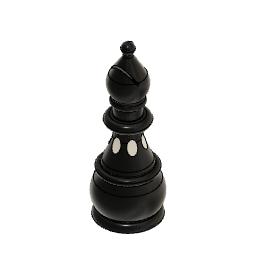
Bishop (Autodesk Fusion 360 design; units mm, degrees)
Autodesk Fusion 360 part; units mm, degrees
(part 1 of 2)
sketch "Bishop" plane through (0, 0, 0) normal (1, 0, 0) x (0, 1, 0)
  spline S0 degree 3 poles (89.633726, 49.908438) (91.318246, 50.120516) (92.983019, 49.910348) (94.642058, 49.967669) knots 0 0 0 0 1 1 1 1
  spline S1 degree 3 poles (94.642058, 49.967669) (95.185947, 49.986137) (95.040743, 49.595738) (95.026729, 49.350542) knots 0 0 0 0 1 1 1 1
  spline S2 degree 3 poles (95.026729, 49.350542) (94.969414, 48.413708) (94.850321, 47.480061) (94.788545, 46.543228) knots 0 0 0 0 1 1 1 1
  spline S3 degree 3 poles (94.788545, 46.543228) (94.752239, 45.984058) (94.746515, 45.546527) (95.629848, 45.661163) knots 0 0 0 0 1 1 1 1
  spline S4 degree 3 poles (95.629848, 45.661163) (96.260983, 45.742682) (96.968548, 45.715933) (97.618789, 45.643968) knots 0 0 0 0 1 1 1 1
  spline S5 degree 3 poles (97.618789, 45.643968) (98.646062, 45.529968) (98.735855, 46.002527) (98.608483, 46.807529) knots 0 0 0 0 1 1 1 1
  spline S6 degree 3 poles (98.608483, 46.807529) (98.484289, 47.590879) (98.454358, 48.390147) (98.321894, 49.171583) knots 0 0 0 0 1 1 1 1
  spline S7 degree 3 poles (98.321894, 49.171583) (98.219993, 49.771514) (98.467098, 49.985501) (99.011618, 49.984864) knots 0 0 0 0 1 1 1 1
  spline S8 degree 3 poles (99.011618, 49.984864) (100.513355, 49.982955) (102.016365, 49.980404) (103.516828, 49.971488) knots 0 0 0 0 1 1 1 1
  spline S9 degree 3 poles (103.516828, 49.971488) (104.025684, 49.968942) (104.316733, 49.857488) (104.202733, 49.195144) knots 0 0 0 0 1 1 1 1
  spline S10 degree 3 poles (104.202733, 49.195144) (103.791319, 46.807524) (103.216226, 44.43328) (101.692197, 42.543053) knots 0 0 0 0 1 1 1 1
  spline S11 degree 3 poles (101.692197, 42.543053) (100.940055, 41.611316) (100.165621, 40.511441) (98.410414, 40.603148) knots 0 0 0 0 1 1 1 1
  spline S12 degree 3 poles (98.410414, 40.603148) (94.261848, 40.819681) (90.094818, 40.657287) (85.935436, 40.638172) knots 0 0 0 0 1 1 1 1
  spline S13 degree 3 poles (85.935436, 40.638172) (85.306206, 40.635626) (84.747673, 40.755991) (84.289127, 41.227277) knots 0 0 0 0 1 1 1 1
  spline S14 degree 3 poles (84.289127, 41.227277) (82.099571, 43.484974) (81.055749, 46.249622) (80.711202, 49.320601) knots 0 0 0 0 1 1 1 1
  spline S15 degree 3 poles (80.711202, 49.320601) (80.677452, 49.61547) (80.535426, 50.020519) (81.126436, 50.01033) knots 0 0 0 0 1 1 1 1
  spline S16 degree 3 poles (81.126436, 50.01033) (82.665752, 49.983581) (84.206331, 49.988037) (85.746278, 49.984218) knots 0 0 0 0 1 1 1 1
  spline S17 degree 3 poles (85.746278, 49.984218) (86.327736, 49.982308) (86.595861, 49.77405) (86.497779, 49.124447) knots 0 0 0 0 1 1 1 1
  spline S18 degree 3 poles (86.497779, 49.124447) (86.358308, 48.198438) (86.310535, 47.258422) (86.213736, 46.326048) knots 0 0 0 0 1 1 1 1
  spline S19 degree 3 poles (86.213736, 46.326048) (86.173611, 45.952208) (86.203542, 45.58346) (86.677374, 45.62995) knots 0 0 0 0 1 1 1 1
  spline S20 degree 3 poles (86.677374, 45.62995) (87.675348, 45.7293) (88.681601, 45.46946) (89.679575, 45.733761) knots 0 0 0 0 1 1 1 1
  spline S21 degree 3 poles (89.679575, 45.733761) (89.932413, 45.80127) (90.126654, 45.768152) (90.090358, 46.115881) knots 0 0 0 0 1 1 1 1
  spline S22 degree 3 poles (90.090358, 46.115881) (89.957884, 47.366698) (90.020933, 48.639794) (89.633726, 49.908438) knots 0 0 0 0 1 1 1 1
  spline S23 degree 3 poles (34.222983, 55.82431) (32.279896, 55.735786) (30.397312, 57.485901) (30.278857, 59.490764) knots 0 0 0 0 1 1 1 1
  spline S24 degree 3 poles (30.278857, 59.490764) (30.143205, 61.784126) (31.853196, 63.806822) (33.99753, 63.887704) knots 0 0 0 0 1 1 1 1
  spline S25 degree 3 poles (33.99753, 63.887704) (36.27115, 63.973046) (38.379183, 62.435008) (38.342882, 59.572919) knots 0 0 0 0 1 1 1 1
  spline S26 degree 3 poles (38.342882, 59.572919) (38.32123, 57.901134) (36.937954, 55.866976) (34.222983, 55.82431) knots 0 0 0 0 1 1 1 1
  spline S27 degree 3 poles (-1.934587, 66.923013) (-1.384334, 66.299521) (-0.785039, 65.859444) (-0.062195, 65.572214) knots 0 0 0 0 1 1 1 1
  spline S28 degree 3 poles (-0.062195, 65.572214) (0.214844, 65.462038) (0.465768, 65.420003) (0.699499, 65.557564) knots 0 0 0 0 1 1 1 1
  spline S29 degree 3 poles (0.699499, 65.557564) (1.023028, 65.7499) (0.936415, 66.105271) (0.871454, 66.378488) knots 0 0 0 0 1 1 1 1
  spline S30 degree 3 poles (0.871454, 66.378488) (0.730069, 66.972686) (0.440932, 67.494281) (-0.037995, 67.904423) knots 0 0 0 0 1 1 1 1
  spline S31 degree 3 poles (-0.037995, 67.904423) (-0.447502, 68.255339) (-0.327771, 68.518998) (0.135233, 68.714521) knots 0 0 0 0 1 1 1 1
  spline S32 degree 3 poles (0.135233, 68.714521) (0.833241, 69.008753) (1.581561, 69.087725) (2.297402, 68.987739) knots 0 0 0 0 1 1 1 1
  spline S33 degree 3 poles (2.297402, 68.987739) (3.616356, 68.80241) (3.670489, 68.565493) (2.908795, 67.495554) knots 0 0 0 0 1 1 1 1
  spline S34 degree 3 poles (2.908795, 67.495554) (2.533045, 66.967589) (1.901268, 66.323077) (2.508206, 65.723151) knots 0 0 0 0 1 1 1 1
  spline S35 degree 3 poles (2.508206, 65.723151) (3.166089, 65.07227) (3.829069, 65.777284) (4.355762, 66.168321) knots 0 0 0 0 1 1 1 1
  spline S36 degree 3 poles (4.355762, 66.168321) (5.255658, 66.836398) (5.526324, 66.817288) (5.709107, 65.735886) knots 0 0 0 0 1 1 1 1
  spline S37 degree 3 poles (5.709107, 65.735886) (5.851765, 64.889487) (5.939017, 64.015066) (5.533331, 63.171217) knots 0 0 0 0 1 1 1 1
  spline S38 degree 3 poles (5.533331, 63.171217) (5.298966, 62.684013) (5.146114, 62.477033) (4.725783, 63.010727) knots 0 0 0 0 1 1 1 1
  spline S39 degree 3 poles (4.725783, 63.010727) (4.343663, 63.494112) (3.809964, 63.806812) (3.2215, 63.971126) knots 0 0 0 0 1 1 1 1
  spline S40 degree 3 poles (3.2215, 63.971126) (2.526038, 64.164735) (2.188499, 63.820189) (2.334344, 63.116447) knots 0 0 0 0 1 1 1 1
  spline S41 degree 3 poles (2.334344, 63.116447) (2.477002, 62.429265) (2.942554, 61.930598) (3.359703, 61.409003) knots 0 0 0 0 1 1 1 1
  spline S42 degree 3 poles (3.359703, 61.409003) (3.68578, 61.001408) (3.646291, 60.814169) (3.095402, 60.672148) knots 0 0 0 0 1 1 1 1
  spline S43 degree 3 poles (3.095402, 60.672148) (2.166847, 60.432049) (1.255489, 60.306587) (0.328207, 60.627567) knots 0 0 0 0 1 1 1 1
  spline S44 degree 3 poles (0.328207, 60.627567) (-0.281913, 60.839008) (-0.651295, 61.066371) (0.018053, 61.712792) knots 0 0 0 0 1 1 1 1
  spline S45 degree 3 poles (0.018053, 61.712792) (0.388711, 62.07071) (0.599512, 62.6025) (0.84853, 63.073781) knots 0 0 0 0 1 1 1 1
  spline S46 degree 3 poles (0.84853, 63.073781) (0.982272, 63.327256) (0.928138, 63.615118) (0.736442, 63.827195) knots 0 0 0 0 1 1 1 1
  spline S47 degree 3 poles (0.736442, 63.827195) (0.536466, 64.048825) (0.28936, 64.049462) (0.004681, 63.928455) knots 0 0 0 0 1 1 1 1
  spline S48 degree 3 poles (0.004681, 63.928455) (-0.576142, 63.68135) (-1.183716, 63.494112) (-1.608507, 62.980159) knots 0 0 0 0 1 1 1 1
  spline S49 degree 3 poles (-1.608507, 62.980159) (-1.946047, 62.571927) (-2.163858, 62.72732) (-2.298236, 63.152112) knots 0 0 0 0 1 1 1 1
  spline S50 degree 3 poles (-2.298236, 63.152112) (-2.696281, 64.412482) (-2.760606, 65.645457) (-1.934587, 66.923013) knots 0 0 0 0 1 1 1 1
  spline S51 degree 3 poles (135.600981, 40.433747) (133.48084, 41.948856) (131.880389, 43.867104) (130.776695, 46.222879) knots 0 0 0 0 1 1 1 1
  spline S52 degree 3 poles (130.776695, 46.222879) (130.465899, 46.885859) (130.146201, 47.600427) (129.560915, 48.05133) knots 0 0 0 0 1 1 1 1
  spline S53 degree 3 poles (129.560915, 48.05133) (128.941889, 48.527708) (128.596692, 48.92957) (128.911938, 49.784249) knots 0 0 0 0 1 1 1 1
  spline S54 degree 3 poles (128.911938, 49.784249) (129.168606, 50.479075) (128.70559, 51.170713) (128.159797, 51.512708) knots 0 0 0 0 1 1 1 1
  spline S55 degree 3 poles (128.159797, 51.512708) (127.687238, 51.80885) (127.289195, 51.243315) (126.961218, 50.86947) knots 0 0 0 0 1 1 1 1
  spline S56 degree 3 poles (126.961218, 50.86947) (126.623037, 50.48544) (126.252379, 50.418567) (125.714224, 50.510274) knots 0 0 0 0 1 1 1 1
  spline S57 degree 3 poles (125.714224, 50.510274) (122.957224, 50.980919) (120.330773, 50.530016) (117.857816, 49.214886) knots 0 0 0 0 1 1 1 1
  spline S58 degree 3 poles (117.857816, 49.214886) (115.538974, 47.98191) (114.006033, 46.068754) (112.929724, 43.706609) knots 0 0 0 0 1 1 1 1
  spline S59 degree 3 poles (112.929724, 43.706609) (111.550267, 40.681484) (110.908306, 37.485043) (110.693678, 34.205806) knots 0 0 0 0 1 1 1 1
  spline S60 degree 3 poles (110.693678, 34.205806) (110.458671, 30.60623) (110.608336, 27.006003) (111.310799, 23.459283) knots 0 0 0 0 1 1 1 1
  spline S61 degree 3 poles (111.310799, 23.459283) (111.687823, 21.556316) (112.158467, 19.674378) (113.022704, 17.900056) knots 0 0 0 0 1 1 1 1
  spline S62 degree 3 poles (113.022704, 17.900056) (113.319487, 17.288026) (113.674859, 16.981059) (114.204092, 16.876611) knots 0 0 0 0 1 1 1 1
  line L0 (114.204092, 16.876611) -> (129.580001, 16.876611)
  spline S63 degree 3 poles (129.580001, 16.876611) (129.992698, 16.962585) (130.1621, 17.234529) (130.216228, 17.738934) knots 0 0 0 0 1 1 1 1
  spline S64 degree 3 poles (130.216228, 17.738934) (130.427028, 19.65846) (130.655028, 21.575431) (130.904037, 23.489223) knots 0 0 0 0 1 1 1 1
  spline S65 degree 3 poles (130.904037, 23.489223) (130.976649, 24.044569) (130.811699, 24.4165) (130.39836, 24.803717) knots 0 0 0 0 1 1 1 1
  spline S66 degree 3 poles (130.39836, 24.803717) (128.511952, 26.564016) (126.765034, 28.446605) (125.529508, 30.746974) knots 0 0 0 0 1 1 1 1
  spline S67 degree 3 poles (125.529508, 30.746974) (124.286984, 33.06326) (123.316386, 35.460438) (123.229139, 38.134652) knots 0 0 0 0 1 1 1 1
  spline S68 degree 3 poles (123.229139, 38.134652) (123.215126, 38.544793) (123.306202, 39.091227) (123.657113, 39.122431) knots 0 0 0 0 1 1 1 1
  spline S69 degree 3 poles (123.657113, 39.122431) (124.127126, 39.164461) (124.017586, 38.584918) (124.08254, 38.246737) knots 0 0 0 0 1 1 1 1
  spline S70 degree 3 poles (124.08254, 38.246737) (124.501593, 36.048902) (125.735215, 35.347079) (127.945149, 35.8795) knots 0 0 0 0 1 1 1 1
  spline S71 degree 3 poles (127.945149, 35.8795) (129.863393, 36.341234) (131.795027, 36.651388) (133.411396, 34.938842) knots 0 0 0 0 1 1 1 1
  spline S72 degree 3 poles (133.411396, 34.938842) (133.62412, 34.713388) (134.325942, 34.094352) (134.890199, 35.017809) knots 0 0 0 0 1 1 1 1
  spline S73 degree 3 poles (134.890199, 35.017809) (135.356383, 35.778231) (135.958228, 36.464135) (136.340995, 37.292066) knots 0 0 0 0 1 1 1 1
  spline S74 degree 3 poles (136.340995, 37.292066) (136.994442, 38.704652) (136.84605, 39.543408) (135.600981, 40.433747) knots 0 0 0 0 1 1 1 1
  line L1 (103.653111, 3.386469) -> (81.020716, 3.386469)
  spline S75 degree 3 poles (81.020716, 3.386469) (80.319525, 3.138091) (79.953959, 2.527966) (79.586489, 1.386061) knots 0 0 0 0 1 1 1 1
  spline S76 degree 3 poles (79.586489, 1.386061) (79.32537, 0.574058) (79.552097, 0.474061) (80.246281, 0.475976) knots 0 0 0 0 1 1 1 1
  spline S77 degree 3 poles (80.246281, 0.475976) (84.005716, 0.489989) (87.76515, 0.489348) (91.523943, 0.486801) knots 0 0 0 0 1 1 1 1
  spline S78 degree 3 poles (91.523943, 0.486801) (95.900499, 0.483614) (100.275151, 0.484887) (104.649802, 0.455597) knots 0 0 0 0 1 1 1 1
  spline S79 degree 3 poles (104.649802, 0.455597) (105.356727, 0.450505) (105.427414, 0.744101) (105.296223, 1.323653) knots 0 0 0 0 1 1 1 1
  spline S80 degree 3 poles (105.296223, 1.323653) (105.024289, 2.521601) (104.542177, 3.152104) (103.653111, 3.386469) knots 0 0 0 0 1 1 1 1
  spline S81 degree 3 poles (40.400605, 16.298341) (40.469388, 16.300256) (40.538171, 16.303434) (40.606949, 16.307262) knots 0 0 0 0 1 1 1 1
  spline S82 degree 3 poles (40.606949, 16.307262) (40.606949, 16.304075) (40.606949, 16.300897) (40.606949, 16.298341) knots 0 0 0 0 1 1 1 1
  line L2 (40.606949, 16.298341) -> (43.205369, 16.298341)
  spline S83 degree 3 poles (43.205369, 16.298341) (43.550556, 17.110986) (42.821339, 17.523674) (42.524556, 18.066921) knots 0 0 0 0 1 1 1 1
  spline S84 degree 3 poles (42.524556, 18.066921) (40.242657, 22.234592) (38.946632, 26.689483) (38.406563, 31.401033) knots 0 0 0 0 1 1 1 1
  spline S85 degree 3 poles (38.406563, 31.401033) (38.28301, 32.48053) (38.38427, 33.596323) (37.99387, 34.750958) knots 0 0 0 0 1 1 1 1
  line L3 (37.99387, 34.750958) -> (30.367372, 34.750958)
  spline S86 degree 3 poles (30.367372, 34.750958) (30.197329, 34.552257) (30.138099, 34.281586) (30.120266, 33.942132) knots 0 0 0 0 1 1 1 1
  spline S87 degree 3 poles (30.120266, 33.942132) (29.969329, 31.074951) (29.496133, 28.251714) (28.833794, 25.461595) knots 0 0 0 0 1 1 1 1
  spline S88 degree 3 poles (28.833794, 25.461595) (28.058724, 22.191279) (26.260209, 19.349569) (24.964184, 16.298332) knots 0 0 0 0 1 1 1 1
  line L4 (24.964184, 16.298332) -> (40.400605, 16.298341)
  spline S89 degree 3 poles (43.658823, 15.93023) (43.592586, 15.93469) (43.496418, 15.932776) (43.403438, 15.936595) knots 0 0 0 0 1 1 1 1
  line L5 (43.403438, 15.936595) -> (24.617728, 15.936595)
  spline S90 degree 3 poles (24.617728, 15.936595) (24.550855, 15.92195) (24.479526, 15.916848) (24.408834, 15.916217) knots 0 0 0 0 1 1 1 1
  spline S91 degree 3 poles (24.408834, 15.916217) (23.657329, 15.90921) (23.370103, 15.344943) (23.40258, 14.792144) knots 0 0 0 0 1 1 1 1
  spline S92 degree 3 poles (23.40258, 14.792144) (23.443978, 14.104966) (23.975126, 13.880144) (24.702429, 13.8827) knots 0 0 0 0 1 1 1 1
  spline S93 degree 3 poles (24.702429, 13.8827) (30.967939, 13.90372) (37.234091, 13.886519) (43.499596, 13.870601) knots 0 0 0 0 1 1 1 1
  spline S94 degree 3 poles (43.499596, 13.870601) (44.129458, 13.869328) (44.707737, 14.011345) (44.789251, 14.695345) knots 0 0 0 0 1 1 1 1
  spline S95 degree 3 poles (44.789251, 14.695345) (44.87779, 15.443667) (44.445997, 15.883739) (43.658823, 15.93023) knots 0 0 0 0 1 1 1 1
  line L6 (84.596094, 37.500329) -> (99.900684, 37.500329)
  spline S96 degree 3 poles (99.900684, 37.500329) (99.965006, 37.507336) (100.028055, 37.513069) (100.091746, 37.523254) knots 0 0 0 0 1 1 1 1
  spline S97 degree 3 poles (100.091746, 37.523254) (100.927957, 37.65254) (101.610674, 38.418053) (101.494128, 39.093132) knots 0 0 0 0 1 1 1 1
  spline S98 degree 3 poles (101.494128, 39.093132) (101.348282, 39.940168) (100.8407, 40.343303) (99.954812, 40.339484) knots 0 0 0 0 1 1 1 1
  spline S99 degree 3 poles (99.954812, 40.339484) (94.996157, 40.314014) (90.037493, 40.303178) (85.079479, 40.303178) knots 0 0 0 0 1 1 1 1
  spline S100 degree 3 poles (85.079479, 40.303178) (84.427324, 40.303178) (83.885351, 40.143961) (83.613407, 39.522379) knots 0 0 0 0 1 1 1 1
  spline S101 degree 3 poles (83.613407, 39.522379) (83.239561, 38.667714) (83.731226, 37.791379) (84.596094, 37.500329) knots 0 0 0 0 1 1 1 1
  spline S102 degree 3 poles (100.648996, 26.139871) (100.282799, 29.357332) (99.991749, 32.579244) (99.687328, 35.801165) knots 0 0 0 0 1 1 1 1
  spline S103 degree 3 poles (99.687328, 35.801165) (99.600082, 36.727168) (99.554223, 37.037964) (99.106503, 37.138592) knots 0 0 0 0 1 1 1 1
  line L7 (99.106503, 37.138592) -> (85.715706, 37.138592)
  spline S104 degree 3 poles (85.715706, 37.138592) (85.515732, 37.069178) (85.367973, 36.90104) (85.336769, 36.489625) knots 0 0 0 0 1 1 1 1
  spline S105 degree 3 poles (85.336769, 36.489625) (85.181371, 34.35102) (84.957831, 32.216875) (84.750851, 30.08273) knots 0 0 0 0 1 1 1 1
  spline S106 degree 3 poles (84.750851, 30.08273) (84.417772, 26.652556) (84.074499, 23.223654) (83.729311, 19.715786) knots 0 0 0 0 1 1 1 1
  spline S107 degree 3 poles (83.729311, 19.715786) (85.568588, 19.715786) (87.440341, 19.718332) (89.313377, 19.715786) knots 0 0 0 0 1 1 1 1
  spline S108 degree 3 poles (89.313377, 19.715786) (92.902769, 19.711966) (96.491519, 19.727884) (100.079638, 19.684582) knots 0 0 0 0 1 1 1 1
  spline S109 degree 3 poles (100.079638, 19.684582) (100.933039, 19.673756) (101.171865, 19.956526) (101.108184, 20.78573) knots 0 0 0 0 1 1 1 1
  spline S110 degree 3 poles (101.108184, 20.78573) (100.972532, 22.572773) (100.850884, 24.372556) (100.648996, 26.139871) knots 0 0 0 0 1 1 1 1
  line L8 (-7.074752, 16.659447) -> (10.456963, 16.659447)
  spline S111 degree 3 poles (10.456963, 16.659447) (10.517466, 17.312874) (10.11178, 17.83447) (9.842387, 18.34524) knots 0 0 0 0 1 1 1 1
  spline S112 degree 3 poles (9.842387, 18.34524) (7.323571, 23.119838) (5.830755, 28.17849) (5.454364, 33.56576) knots 0 0 0 0 1 1 1 1
  spline S113 degree 3 poles (5.454364, 33.56576) (5.356923, 34.963691) (5.328902, 35.233079) (4.406717, 35.35154) knots 0 0 0 0 1 1 1 1
  line L9 (4.406717, 35.35154) -> (-2.121826, 35.35154)
  spline S114 degree 3 poles (-2.121826, 35.35154) (-2.345368, 35.289763) (-2.523053, 35.143286) (-2.524963, 34.788546) knots 0 0 0 0 1 1 1 1
  spline S115 degree 3 poles (-2.524963, 34.788546) (-2.526873, 34.251665) (-2.703285, 33.723063) (-2.713477, 33.210388) knots 0 0 0 0 1 1 1 1
  spline S116 degree 3 poles (-2.713477, 33.210388) (-2.769522, 30.417724) (-3.357352, 27.719312) (-4.028609, 25.031727) knots 0 0 0 0 1 1 1 1
  spline S117 degree 3 poles (-4.028609, 25.031727) (-4.667387, 22.475332) (-5.93603, 20.165411) (-6.91044, 17.740858) knots 0 0 0 0 1 1 1 1
  spline S118 degree 3 poles (-6.91044, 17.740858) (-7.072842, 17.337072) (-7.354973, 16.930118) (-7.074752, 16.659447) knots 0 0 0 0 1 1 1 1
  line L10 (-7.923698, 14.23298) -> (11.334566, 14.23298)
  spline S119 degree 3 poles (11.334566, 14.23298) (11.694399, 14.381371) (11.9294, 14.711272) (11.997547, 15.125233) knots 0 0 0 0 1 1 1 1
  spline S120 degree 3 poles (11.997547, 15.125233) (12.087981, 15.680578) (11.543461, 16.099641) (10.931427, 16.267779) knots 0 0 0 0 1 1 1 1
  spline S121 degree 3 poles (10.931427, 16.267779) (10.855001, 16.28943) (10.743552, 16.279878) (10.646747, 16.29771) knots 0 0 0 0 1 1 1 1
  line L11 (10.646747, 16.29771) -> (-7.513554, 16.29771)
  spline S122 degree 3 poles (-7.513554, 16.29771) (-7.530113, 16.295795) (-7.547309, 16.295164) (-7.564504, 16.293891) knots 0 0 0 0 1 1 1 1
  spline S123 degree 3 poles (-7.564504, 16.293891) (-8.289261, 16.249305) (-8.71023, 15.827065) (-8.68985, 15.139246) knots 0 0 0 0 1 1 1 1
  spline S124 degree 3 poles (-8.68985, 15.139246) (-8.673293, 14.611276) (-8.379059, 14.328506) (-7.923698, 14.23298) knots 0 0 0 0 1 1 1 1
  line L12 (-8.959882, 3.332341) -> (11.658098, 3.332341)
  spline S125 degree 3 poles (11.658098, 3.332341) (12.099448, 3.436147) (12.418519, 3.694719) (12.675177, 4.216315) knots 0 0 0 0 1 1 1 1
  spline S126 degree 3 poles (12.675177, 4.216315) (14.000501, 6.905173) (13.597361, 9.489585) (12.241469, 11.99566) knots 0 0 0 0 1 1 1 1
  spline S127 degree 3 poles (12.241469, 11.99566) (11.889917, 12.645269) (11.711594, 13.533693) (10.995117, 13.871243) knots 0 0 0 0 1 1 1 1
  line L13 (10.995117, 13.871243) -> (-2.595655, 13.871243)
  spline S128 degree 3 poles (-2.595655, 13.871243) (-3.303216, 13.849591) (-4.010141, 13.836851) (-4.71197, 13.871243) knots 0 0 0 0 1 1 1 1
  line L14 (-4.71197, 13.871243) -> (-7.158818, 13.871243)
  spline S129 degree 3 poles (-7.158818, 13.871243) (-8.159338, 13.627325) (-8.875179, 12.948417) (-9.496763, 11.777854) knots 0 0 0 0 1 1 1 1
  spline S130 degree 3 poles (-9.496763, 11.777854) (-10.889595, 9.154591) (-10.999137, 6.645969) (-9.687823, 4.015699) knots 0 0 0 0 1 1 1 1
  spline S131 degree 3 poles (-9.687823, 4.015699) (-9.501221, 3.639308) (-9.270036, 3.427867) (-8.959882, 3.332341) knots 0 0 0 0 1 1 1 1
  line L15 (11.927491, 2.972509) -> (-8.987267, 2.972509)
  spline S132 degree 3 poles (-8.987267, 2.972509) (-9.875698, 2.803739) (-10.470532, 2.010199) (-10.318322, 0.98866) knots 0 0 0 0 1 1 1 1
  spline S133 degree 3 poles (-10.318322, 0.98866) (-10.169294, -0.020139) (-9.281501, 0.614815) (-8.733794, 0.482982) knots 0 0 0 0 1 1 1 1
  spline S134 degree 3 poles (-8.733794, 0.482982) (-8.576486, 0.443499) (-8.401349, 0.474703) (-8.233852, 0.474703) knots 0 0 0 0 1 1 1 1
  spline S135 degree 3 poles (-8.233852, 0.474703) (-1.544824, 0.472788) (5.145482, 0.463877) (11.835147, 0.494449) knots 0 0 0 0 1 1 1 1
  spline S136 degree 3 poles (11.835147, 0.494449) (12.251659, 0.496364) (12.866239, 0.196393) (13.108884, 0.730729) knots 0 0 0 0 1 1 1 1
  spline S137 degree 3 poles (13.108884, 0.730729) (13.357262, 1.276522) (13.06494, 1.832509) (12.776437, 2.343278) knots 0 0 0 0 1 1 1 1
  spline S138 degree 3 poles (12.776437, 2.343278) (12.559904, 2.726035) (12.268218, 2.897992) (11.927491, 2.972509) knots 0 0 0 0 1 1 1 1
  line L16 (54.497685, 15.697138) -> (71.435844, 15.697138)
  spline S139 degree 3 poles (71.435844, 15.697138) (72.074626, 15.923864) (72.335104, 16.453098) (72.172699, 17.042845) knots 0 0 0 0 1 1 1 1
  spline S140 degree 3 poles (72.172699, 17.042845) (72.007117, 17.643407) (71.491886, 17.970763) (70.777324, 17.964397) knots 0 0 0 0 1 1 1 1
  spline S141 degree 3 poles (70.777324, 17.964397) (67.759205, 17.9402) (64.740445, 17.954203) (61.721695, 17.956118) knots 0 0 0 0 1 1 1 1
  spline S142 degree 3 poles (61.721695, 17.956118) (59.507942, 17.956759) (57.294188, 17.968216) (55.080435, 17.963124) knots 0 0 0 0 1 1 1 1
  spline S143 degree 3 poles (55.080435, 17.963124) (54.254418, 17.960578) (53.827076, 17.47146) (53.825803, 16.695753) knots 0 0 0 0 1 1 1 1
  spline S144 degree 3 poles (53.825803, 16.695753) (53.823879, 16.138493) (54.08181, 15.827055) (54.497685, 15.697138) knots 0 0 0 0 1 1 1 1
  line L17 (82.414818, 16.902092) -> (83.703841, 16.902092)
  spline S145 degree 3 poles (83.703841, 16.902092) (83.718486, 16.902092) (83.732499, 16.902092) (83.747144, 16.902092) knots 0 0 0 0 1 1 1 1
  line L18 (83.747144, 16.902092) -> (102.137993, 16.902092)
  spline S146 degree 3 poles (102.137993, 16.902092) (103.056358, 17.005266) (103.557575, 17.431967) (103.529549, 18.091128) knots 0 0 0 0 1 1 1 1
  spline S147 degree 3 poles (103.529549, 18.091128) (103.495158, 18.902499) (102.855102, 19.346391) (101.710019, 19.35022) knots 0 0 0 0 1 1 1 1
  spline S148 degree 3 poles (101.710019, 19.35022) (100.208924, 19.356585) (98.706546, 19.357858) (97.20545, 19.361687) knots 0 0 0 0 1 1 1 1
  spline S149 degree 3 poles (97.20545, 19.361687) (93.57021, 19.368052) (89.935601, 19.378246) (86.299709, 19.379519) knots 0 0 0 0 1 1 1 1
  spline S150 degree 3 poles (86.299709, 19.379519) (85.202381, 19.381434) (84.106334, 19.361687) (83.009015, 19.348947) knots 0 0 0 0 1 1 1 1
  spline S151 degree 3 poles (83.009015, 19.348947) (82.125041, 19.338121) (81.688788, 18.765575) (81.683055, 18.004522) knots 0 0 0 0 1 1 1 1
  spline S152 degree 3 poles (81.683055, 18.004522) (81.678594, 17.44598) (81.924426, 17.047296) (82.414818, 16.902092) knots 0 0 0 0 1 1 1 1
  spline S153 degree 3 poles (105.175858, 11.831351) (104.562556, 13.336907) (103.625085, 14.64695) (102.860204, 16.059516) knots 0 0 0 0 1 1 1 1
  spline S154 degree 3 poles (102.860204, 16.059516) (102.627111, 16.490036) (102.236707, 16.519976) (101.822746, 16.519335) knots 0 0 0 0 1 1 1 1
  spline S155 degree 3 poles (101.822746, 16.519335) (100.650269, 16.519335) (99.477161, 16.518694) (98.304684, 16.518694) knots 0 0 0 0 1 1 1 1
  spline S156 degree 3 poles (98.304684, 16.518694) (97.187618, 16.518052) (96.071184, 16.518694) (94.954759, 16.518694) knots 0 0 0 0 1 1 1 1
  spline S157 degree 3 poles (94.954759, 16.518694) (94.954759, 16.526332) (94.954759, 16.532707) (94.954759, 16.540345) knots 0 0 0 0 1 1 1 1
  line L19 (94.954759, 16.540345) -> (83.143394, 16.540345)
  spline S158 degree 3 poles (83.143394, 16.540345) (82.995643, 16.509773) (82.863811, 16.44099) (82.759364, 16.288147) knots 0 0 0 0 1 1 1 1
  spline S159 degree 3 poles (82.759364, 16.288147) (81.742285, 14.800424) (80.672351, 13.33372) (79.815762, 11.754279) knots 0 0 0 0 1 1 1 1
  spline S160 degree 3 poles (79.815762, 11.754279) (78.76811, 9.821381) (79.145775, 7.766845) (79.850785, 5.816756) knots 0 0 0 0 1 1 1 1
  spline S161 degree 3 poles (79.850785, 5.816756) (80.337989, 4.468502) (80.64687, 3.983213) (81.492634, 3.83864) knots 0 0 0 0 1 1 1 1
  line L20 (81.492634, 3.83864) -> (103.706608, 3.83864)
  spline S162 degree 3 poles (103.706608, 3.83864) (103.921868, 3.920795) (104.117391, 4.075552) (104.274062, 4.357048) knots 0 0 0 0 1 1 1 1
  spline S163 degree 3 poles (104.274062, 4.357048) (105.591102, 6.723022) (106.268085, 9.150772) (105.175858, 11.831351) knots 0 0 0 0 1 1 1 1
  spline S164 degree 3 poles (44.687369, 3.21388) (45.687889, 3.592818) (45.880856, 4.682499) (46.142616, 5.61615) knots 0 0 0 0 1 1 1 1
  spline S165 degree 3 poles (46.142616, 5.61615) (46.897944, 8.312647) (45.866211, 10.664608) (44.542165, 12.940137) knots 0 0 0 0 1 1 1 1
  spline S166 degree 3 poles (44.542165, 12.940137) (44.21481, 13.503762) (43.835882, 13.66744) (43.172902, 13.663621) knots 0 0 0 0 1 1 1 1
  spline S167 degree 3 poles (43.172902, 13.663621) (37.064058, 13.629229) (30.955218, 13.632417) (24.846374, 13.671901) knots 0 0 0 0 1 1 1 1
  spline S168 degree 3 poles (24.846374, 13.671901) (24.241351, 13.67572) (23.848401, 13.465552) (23.602569, 13.025479) knots 0 0 0 0 1 1 1 1
  spline S169 degree 3 poles (23.602569, 13.025479) (23.094986, 12.114762) (22.40844, 11.323127) (22.015494, 10.328983) knots 0 0 0 0 1 1 1 1
  spline S170 degree 3 poles (22.015494, 10.328983) (20.998415, 7.757943) (21.449318, 5.432736) (22.900105, 3.21389) knots 0 0 0 0 1 1 1 1
  line L21 (22.900105, 3.21389) -> (44.687369, 3.21388)
  line L22 (44.939566, 2.851502) -> (22.799472, 2.851502)
  spline S171 degree 3 poles (22.799472, 2.851502) (22.635157, 2.717755) (22.463205, 2.577653) (22.298254, 2.426074) knots 0 0 0 0 1 1 1 1
  spline S172 degree 3 poles (22.298254, 2.426074) (21.798952, 1.970074) (21.665205, 1.312196) (21.841618, 0.762574) knots 0 0 0 0 1 1 1 1
  spline S173 degree 3 poles (21.841618, 0.762574) (22.010388, 0.233341) (22.663815, 0.504002) (23.095613, 0.499551) knots 0 0 0 0 1 1 1 1
  spline S174 degree 3 poles (23.095613, 0.499551) (25.97362, 0.471525) (28.851631, 0.468979) (31.730275, 0.472798) knots 0 0 0 0 1 1 1 1
  spline S175 degree 3 poles (31.730275, 0.472798) (36.262865, 0.479163) (40.794824, 0.513555) (45.326783, 0.488716) knots 0 0 0 0 1 1 1 1
  spline S176 degree 3 poles (45.326783, 0.488716) (46.156619, 0.483624) (46.136882, 0.768298) (46.033708, 1.444019) knots 0 0 0 0 1 1 1 1
  spline S177 degree 3 poles (46.033708, 1.444019) (45.909523, 2.263038) (45.499372, 2.646426) (44.939566, 2.851502) knots 0 0 0 0 1 1 1 1
  line L23 (113.152, 14.427861) -> (130.611103, 14.427861)
  spline S178 degree 3 poles (130.611103, 14.427861) (131.033343, 14.69344) (131.374711, 15.049443) (131.150521, 15.695864) knots 0 0 0 0 1 1 1 1
  spline S179 degree 3 poles (131.150521, 15.695864) (130.874126, 16.491309) (130.188221, 16.533348) (129.495942, 16.532075) knots 0 0 0 0 1 1 1 1
  spline S180 degree 3 poles (129.495942, 16.532075) (129.360922, 16.532075) (129.227826, 16.526983) (129.092807, 16.528256) knots 0 0 0 0 1 1 1 1
  spline S181 degree 3 poles (129.092807, 16.528256) (125.747965, 16.532075) (122.401869, 16.542269) (119.056395, 16.540355) knots 0 0 0 0 1 1 1 1
  spline S182 degree 3 poles (119.056395, 16.540355) (117.313287, 16.539713) (115.570178, 16.514243) (113.827069, 16.509782) knots 0 0 0 0 1 1 1 1
  spline S183 degree 3 poles (113.827069, 16.509782) (113.039263, 16.509141) (112.466086, 16.15823) (112.461625, 15.361512) knots 0 0 0 0 1 1 1 1
  spline S184 degree 3 poles (112.461625, 15.361512) (112.459089, 14.826536) (112.748865, 14.55396) (113.152, 14.427861) knots 0 0 0 0 1 1 1 1
  spline S185 degree 3 poles (130.700915, 3.0069) (129.637978, 3.006259) (128.57504, 3.0069) (127.512122, 3.0069) knots 0 0 0 0 1 1 1 1
  spline S186 degree 3 poles (127.512122, 3.0069) (127.512122, 3.009446) (127.512122, 3.010719) (127.512122, 3.013265) knots 0 0 0 0 1 1 1 1
  line L24 (127.512122, 3.013265) -> (115.394421, 3.013265)
  spline S187 degree 3 poles (115.394421, 3.013265) (114.960714, 2.982693) (114.527648, 2.957222) (114.099033, 3.013265) knots 0 0 0 0 1 1 1 1
  line L25 (114.099033, 3.013265) -> (112.699197, 3.013265)
  spline S188 degree 3 poles (112.699197, 3.013265) (112.645059, 3.003071) (112.584566, 3.003071) (112.51896, 3.013265) knots 0 0 0 0 1 1 1 1
  line L26 (112.517687, 3.013265) -> (112.114552, 3.013265)
  spline S189 degree 3 poles (112.114552, 3.013265) (111.578944, 2.922831) (111.299362, 2.45792) (111.075822, 1.994913) knots 0 0 0 0 1 1 1 1
  spline S190 degree 3 poles (111.075822, 1.994913) (110.566967, 0.94663) (110.911513, 0.468338) (112.064243, 0.492545) knots 0 0 0 0 1 1 1 1
  spline S191 degree 3 poles (112.064243, 0.492545) (112.59921, 0.504643) (113.134819, 0.491903) (113.670427, 0.491903) knots 0 0 0 0 1 1 1 1
  spline S192 degree 3 poles (113.670427, 0.491903) (119.632158, 0.488716) (125.595161, 0.48617) (131.557523, 0.488716) knots 0 0 0 0 1 1 1 1
  spline S193 degree 3 poles (131.557523, 0.488716) (131.872129, 0.489357) (132.237695, 0.390634) (132.353609, 0.87466) knots 0 0 0 0 1 1 1 1
  spline S194 degree 3 poles (132.353609, 0.87466) (132.591132, 1.861167) (131.714175, 3.008805) (130.700915, 3.0069) knots 0 0 0 0 1 1 1 1
  line L27 (130.456356, 14.066114) -> (113.343704, 14.066114)
  spline S195 degree 3 poles (113.343704, 14.066114) (112.922095, 13.868687) (112.611309, 13.455358) (112.306247, 12.964966) knots 0 0 0 0 1 1 1 1
  spline S196 degree 3 poles (112.306247, 12.964966) (111.975072, 12.432545) (111.719687, 11.875917) (111.439473, 11.326305) knots 0 0 0 0 1 1 1 1
  spline S197 degree 3 poles (111.439473, 11.326305) (110.242158, 8.99346) (110.368256, 6.663792) (111.416549, 4.3112) knots 0 0 0 0 1 1 1 1
  spline S198 degree 3 poles (111.416549, 4.3112) (111.624171, 3.843101) (111.871276, 3.50492) (112.236832, 3.375002) knots 0 0 0 0 1 1 1 1
  line L28 (112.236832, 3.375002) -> (113.013171, 3.375002)
  spline S199 degree 3 poles (113.013171, 3.375002) (113.016358, 3.375002) (113.019536, 3.376275) (113.020809, 3.376917) knots 0 0 0 0 1 1 1 1
  spline S200 degree 3 poles (113.020809, 3.376917) (113.021451, 3.377558) (113.021451, 3.379463) (113.021451, 3.380736) knots 0 0 0 0 1 1 1 1
  spline S201 degree 3 poles (113.021451, 3.380736) (113.024638, 3.379463) (113.026543, 3.377548) (113.028457, 3.376917) knots 0 0 0 0 1 1 1 1
  spline S202 degree 3 poles (113.028457, 3.376917) (114.292, 3.376917) (115.555553, 3.376917) (116.819095, 3.376917) knots 0 0 0 0 1 1 1 1
  spline S203 degree 2 poles (116.819095, 3.376917) (116.819095, 3.376275) (116.819095, 3.375002) knots 0 0 0 1 1 1
  line L29 (116.819095, 3.375002) -> (131.058201, 3.375002)
  spline S204 degree 3 poles (131.058201, 3.375002) (131.351155, 3.46289) (131.563879, 3.659686) (131.721172, 3.976206) knots 0 0 0 0 1 1 1 1
  spline S205 degree 3 poles (131.721172, 3.976206) (132.186715, 4.907311) (132.57331, 5.850506) (132.654182, 6.925542) knots 0 0 0 0 1 1 1 1
  spline S206 degree 3 poles (132.654182, 6.925542) (132.852892, 9.594032) (131.860642, 11.85618) (130.456356, 14.066114) knots 0 0 0 0 1 1 1 1
  line L30 (113.020168, 3.376918) -> (113.020168, 3.375008)
  line L31 (113.020168, 3.375008) -> (113.030995, 3.375008)
  line L32 (113.030995, 3.375008) -> (113.027174, 3.376918)
  line L33 (113.027174, 3.376918) -> (113.020809, 3.376917)
  line L34 (113.020809, 3.376917) -> (113.020168, 3.376918)
  spline S207 degree 3 poles (67.892942, 40.107033) (67.408284, 40.542014) (67.601261, 40.706964) (67.860465, 41.123471) knots 0 0 0 0 1 1 1 1
  spline S208 degree 3 poles (67.860465, 41.123471) (69.239281, 43.336593) (69.754511, 45.614032) (68.39034, 48.081897) knots 0 0 0 0 1 1 1 1
  spline S209 degree 3 poles (68.39034, 48.081897) (67.209584, 50.217952) (65.881077, 52.248927) (64.422652, 54.199021) knots 0 0 0 0 1 1 1 1
  spline S210 degree 3 poles (64.422652, 54.199021) (64.207393, 54.48561) (64.090846, 54.714246) (64.162175, 54.98173) knots 0 0 0 0 1 1 1 1
  spline S211 degree 3 poles (64.162175, 54.98173) (64.723254, 55.348564) (65.095185, 55.981613) (65.095185, 56.70255) knots 0 0 0 0 1 1 1 1
  spline S212 degree 3 poles (65.095185, 56.70255) (65.095185, 57.838085) (64.175547, 58.75836) (63.039376, 58.75836) knots 0 0 0 0 1 1 1 1
  spline S213 degree 3 poles (63.039376, 58.75836) (61.903205, 58.75836) (60.983567, 57.838085) (60.983567, 56.70255) knots 0 0 0 0 1 1 1 1
  spline S214 degree 3 poles (60.983567, 56.70255) (60.983567, 55.986073) (61.351037, 55.355575) (61.906392, 54.9881) knots 0 0 0 0 1 1 1 1
  spline S215 degree 3 poles (61.906392, 54.9881) (61.957343, 54.521911) (61.631261, 54.146161) (61.323021, 53.71946) knots 0 0 0 0 1 1 1 1
  spline S216 degree 3 poles (61.323021, 53.71946) (61.087382, 53.393383) (60.865116, 53.055206) (60.604629, 52.749507) knots 0 0 0 0 1 1 1 1
  spline S217 degree 3 poles (60.604629, 52.749507) (60.063929, 52.1171) (59.972221, 51.495512) (60.397008, 50.729363) knots 0 0 0 0 1 1 1 1
  spline S218 degree 3 poles (60.397008, 50.729363) (60.865106, 49.88169) (61.217932, 48.967785) (61.603876, 48.075532) knots 0 0 0 0 1 1 1 1
  spline S219 degree 3 poles (60.992478, 47.803593) (60.898856, 47.980642) (60.851093, 48.185076) (60.746646, 48.355756) knots 0 0 0 0 1 1 1 1
  spline S220 degree 3 poles (60.746646, 48.355756) (60.26708, 49.134645) (60.123149, 50.100774) (59.451889, 50.816614) knots 0 0 0 0 1 1 1 1
  spline S221 degree 3 poles (59.451889, 50.816614) (59.097149, 50.358068) (58.735412, 49.996963) (58.50232, 49.566443) knots 0 0 0 0 1 1 1 1
  spline S222 degree 3 poles (58.50232, 49.566443) (57.756544, 48.186349) (56.696162, 46.963563) (56.829267, 45.188609) knots 0 0 0 0 1 1 1 1
  spline S223 degree 3 poles (56.829267, 45.188609) (56.950274, 43.592619) (57.493521, 42.217622) (58.360935, 40.929231) knots 0 0 0 0 1 1 1 1
  spline S224 degree 3 poles (58.360935, 40.929231) (58.498501, 40.725428) (58.650711, 40.605063) (58.466656, 40.330573) knots 0 0 0 0 1 1 1 1
  spline S225 degree 3 poles (58.466656, 40.330573) (57.66229, 39.131984) (57.680123, 38.581731) (58.853231, 38.207254) knots 0 0 0 0 1 1 1 1
  line L35 (58.853231, 38.207254) -> (67.445863, 38.207254)
  spline S226 degree 3 poles (67.445863, 38.207254) (67.458603, 38.211714) (67.470061, 38.215533) (67.481528, 38.221267) knots 0 0 0 0 1 1 1 1
  spline S227 degree 3 poles (67.481528, 38.221267) (68.360409, 38.661339) (68.590955, 39.48099) (67.892942, 40.107033) knots 0 0 0 0 1 1 1 1
  line L36 (53.937247, 3.574986) -> (71.608432, 3.574986)
  spline S228 degree 3 poles (71.608432, 3.574986) (72.052334, 3.669239) (72.349107, 3.928443) (72.596854, 4.430933) knots 0 0 0 0 1 1 1 1
  spline S229 degree 3 poles (72.596854, 4.430933) (73.989683, 7.257989) (74.014521, 10.044289) (72.620419, 12.887272) knots 0 0 0 0 1 1 1 1
  spline S230 degree 3 poles (72.620419, 12.887272) (72.221735, 13.70119) (71.628811, 14.435499) (71.4091, 15.335391) knots 0 0 0 0 1 1 1 1
  line L37 (71.4091, 15.335391) -> (56.537586, 15.335391)
  spline S231 degree 3 poles (56.537586, 15.335391) (56.471991, 15.328384) (56.408942, 15.328384) (56.345892, 15.335391) knots 0 0 0 0 1 1 1 1
  line L38 (56.345892, 15.335391) -> (55.149218, 15.335391)
  spline S232 degree 3 poles (55.149218, 15.335391) (54.367145, 15.106759) (53.927063, 14.373082) (53.437313, 13.51522) knots 0 0 0 0 1 1 1 1
  spline S233 degree 3 poles (53.437313, 13.51522) (51.761073, 10.578614) (51.602497, 7.657305) (52.948195, 4.592055) knots 0 0 0 0 1 1 1 1
  spline S234 degree 3 poles (52.948195, 4.592055) (53.18256, 4.057729) (53.462774, 3.697265) (53.937247, 3.574986) knots 0 0 0 0 1 1 1 1
  line L39 (71.827521, 3.21388) -> (59.138557, 3.21388)
  spline S235 degree 3 poles (59.138557, 3.21388) (58.790192, 3.183949) (58.431632, 3.163571) (58.072442, 3.21388) knots 0 0 0 0 1 1 1 1
  line L40 (58.072442, 3.21388) -> (54.089468, 3.21388)
  spline S236 degree 3 poles (54.089468, 3.21388) (53.050096, 3.068035) (52.639323, 2.60567) (52.510668, 1.434466) knots 0 0 0 0 1 1 1 1
  spline S237 degree 3 poles (52.510668, 1.434466) (52.438698, 0.769571) (52.595369, 0.483624) (53.369172, 0.489989) knots 0 0 0 0 1 1 1 1
  spline S238 degree 3 poles (53.369172, 0.489989) (57.312021, 0.52438) (61.256784, 0.488074) (65.200916, 0.485528) knots 0 0 0 0 1 1 1 1
  spline S239 degree 3 poles (65.200916, 0.485528) (67.577073, 0.482982) (69.955136, 0.493808) (72.330662, 0.504002) knots 0 0 0 0 1 1 1 1
  spline S240 degree 3 poles (72.330662, 0.504002) (72.645909, 0.504643) (72.994284, 0.395736) (73.095544, 0.910966) knots 0 0 0 0 1 1 1 1
  spline S241 degree 3 poles (73.095544, 0.910966) (73.282127, 1.861167) (72.694294, 2.917739) (71.827521, 3.21388) knots 0 0 0 0 1 1 1 1
  spline S242 degree 3 poles (41.389663, 55.020582) (40.145857, 54.344866) (38.920525, 54.257614) (37.769704, 55.001476) knots 0 0 0 0 1 1 1 1
  spline S243 degree 3 poles (37.769704, 55.001476) (37.085709, 55.443463) (36.671107, 55.404616) (35.989658, 55.011665) knots 0 0 0 0 1 1 1 1
  spline S244 degree 3 poles (35.989658, 55.011665) (34.79362, 54.3213) (33.516696, 54.011782) (32.260154, 55.061343) knots 0 0 0 0 1 1 1 1
  spline S245 degree 3 poles (32.260154, 55.061343) (31.965286, 55.307812) (31.543677, 55.640254) (30.999153, 55.274057) knots 0 0 0 0 1 1 1 1
  spline S246 degree 3 poles (30.999153, 55.274057) (29.612689, 54.342957) (28.179735, 54.322573) (26.688829, 55.118022) knots 0 0 0 0 1 1 1 1
  spline S247 degree 3 poles (26.688829, 55.118022) (25.636722, 55.679101) (24.617733, 55.305261) (23.940103, 54.235958) knots 0 0 0 0 1 1 1 1
  spline S248 degree 3 poles (23.940103, 54.235958) (23.427424, 53.42841) (23.622305, 52.319619) (24.492903, 51.634988) knots 0 0 0 0 1 1 1 1
  spline S249 degree 3 poles (24.492903, 51.634988) (27.952371, 48.913647) (29.136947, 45.105813) (29.567472, 40.968073) knots 0 0 0 0 1 1 1 1
  spline S250 degree 3 poles (29.567472, 40.968073) (29.687205, 39.815343) (29.698031, 39.370168) (29.247128, 39.183566) knots 0 0 0 0 1 1 1 1
  line L41 (29.247128, 39.183566) -> (27.424411, 39.183566)
  spline S251 degree 3 poles (27.424411, 39.183566) (26.299702, 39.183566) (25.387707, 38.271566) (25.387707, 37.147494) knots 0 0 0 0 1 1 1 1
  spline S252 degree 3 poles (25.387707, 37.147494) (25.387707, 36.084556) (26.202261, 35.212691) (27.240996, 35.119701) knots 0 0 0 0 1 1 1 1
  spline S253 degree 3 poles (27.240996, 35.119701) (27.253095, 35.117787) (27.265199, 35.113968) (27.277297, 35.11078) knots 0 0 0 0 1 1 1 1
  line L42 (27.277297, 35.11078) -> (27.424416, 35.11078)
  line L43 (27.424416, 35.11078) -> (40.364946, 35.11078)
  line L44 (40.364946, 35.11078) -> (40.419716, 35.11078)
  spline S254 degree 3 poles (40.419716, 35.11078) (40.429905, 35.112053) (40.438821, 35.113968) (40.448374, 35.115241) knots 0 0 0 0 1 1 1 1
  spline S255 degree 3 poles (40.448374, 35.115241) (40.826675, 35.130527) (41.178227, 35.247704) (41.476278, 35.442596) knots 0 0 0 0 1 1 1 1
  spline S256 degree 3 poles (41.476278, 35.442596) (41.832923, 35.648944) (42.088944, 35.936165) (42.206768, 36.283898) knots 0 0 0 0 1 1 1 1
  spline S257 degree 3 poles (42.206768, 36.283898) (42.330316, 36.54629) (42.401013, 36.838612) (42.401013, 37.147494) knots 0 0 0 0 1 1 1 1
  spline S258 degree 3 poles (42.401013, 37.147494) (42.401013, 38.272208) (41.489655, 39.183566) (40.364946, 39.183566) knots 0 0 0 0 1 1 1 1
  line L45 (40.364946, 39.183566) -> (38.854293, 39.183566)
  spline S259 degree 3 poles (38.854293, 39.183566) (38.677244, 39.348517) (38.688706, 39.68351) (38.714181, 40.364323) knots 0 0 0 0 1 1 1 1
  spline S260 degree 3 poles (38.714181, 40.364323) (38.716727, 40.431191) (38.707174, 40.498701) (38.710998, 40.564938) knots 0 0 0 0 1 1 1 1
  spline S261 degree 3 poles (38.710998, 40.564938) (38.985489, 44.859339) (40.256679, 48.698382) (43.678569, 51.582123) knots 0 0 0 0 1 1 1 1
  spline S262 degree 3 poles (43.678569, 51.582123) (44.122471, 51.955963) (44.554905, 52.40623) (44.574642, 53.08386) knots 0 0 0 0 1 1 1 1
  spline S263 degree 3 poles (44.574642, 53.08386) (44.624951, 54.844169) (42.985658, 55.887996) (41.389663, 55.020582) knots 0 0 0 0 1 1 1 1
  line L46 (-32.399826, 13.155397) -> (-15.644454, 13.155397)
  spline S264 degree 3 poles (-15.644454, 13.155397) (-15.247685, 13.321621) (-14.95982, 13.618404) (-15.063631, 14.127891) knots 0 0 0 0 1 1 1 1
  spline S265 degree 3 poles (-15.063631, 14.127891) (-15.168079, 14.641207) (-15.42601, 14.869207) (-15.755908, 14.973654) knots 0 0 0 0 1 1 1 1
  line L47 (-15.755908, 14.973654) -> (-32.171827, 14.973654)
  spline S266 degree 3 poles (-32.171827, 14.973654) (-32.570507, 14.801697) (-32.775578, 14.430407) (-32.787042, 13.883973) knots 0 0 0 0 1 1 1 1
  spline S267 degree 3 poles (-32.787042, 13.883973) (-32.795958, 13.461733) (-32.638652, 13.255384) (-32.399826, 13.155397) knots 0 0 0 0 1 1 1 1
  line L48 (-32.990203, 3.078229) -> (-15.071272, 3.078229)
  spline S268 degree 3 poles (-15.071272, 3.078229) (-14.584704, 3.358453) (-14.343969, 3.928453) (-14.108326, 4.518821) knots 0 0 0 0 1 1 1 1
  spline S269 degree 3 poles (-14.108326, 4.518821) (-13.337079, 6.44344) (-13.590552, 8.332394) (-14.347152, 10.174848) knots 0 0 0 0 1 1 1 1
  spline S270 degree 3 poles (-14.347152, 10.174848) (-14.733093, 11.114864) (-15.12859, 12.074628) (-15.900473, 12.793651) knots 0 0 0 0 1 1 1 1
  line L49 (-15.900473, 12.793651) -> (-32.182017, 12.793651)
  spline S271 degree 3 poles (-32.182017, 12.793651) (-32.238698, 12.761174) (-32.291558, 12.718503) (-32.338687, 12.656085) knots 0 0 0 0 1 1 1 1
  spline S272 degree 3 poles (-32.338687, 12.656085) (-34.116823, 10.28948) (-35.260002, 7.771937) (-34.172231, 4.741088) knots 0 0 0 0 1 1 1 1
  spline S273 degree 3 poles (-34.172231, 4.741088) (-33.792657, 3.683252) (-33.569753, 3.249545) (-32.990203, 3.078229) knots 0 0 0 0 1 1 1 1
  line L50 (-15.023506, 2.717124) -> (-33.33029, 2.717124)
  spline S274 degree 3 poles (-33.33029, 2.717124) (-33.992634, 2.501864) (-34.375391, 1.840788) (-34.297057, 1.011594) knots 0 0 0 0 1 1 1 1
  spline S275 degree 3 poles (-34.297057, 1.011594) (-34.209169, 0.079216) (-33.451932, 0.507831) (-33.041789, 0.502739) knots 0 0 0 0 1 1 1 1
  spline S276 degree 3 poles (-33.041789, 0.502739) (-29.359415, 0.460068) (-25.676406, 0.48236) (-21.994031, 0.486179) knots 0 0 0 0 1 1 1 1
  spline S277 degree 3 poles (-21.994031, 0.486179) (-19.524892, 0.487453) (-17.054479, 0.507199) (-14.585341, 0.486179) knots 0 0 0 0 1 1 1 1
  spline S278 degree 3 poles (-14.585341, 0.486179) (-13.970126, 0.479814) (-13.839567, 0.689982) (-13.965032, 1.262518) knots 0 0 0 0 1 1 1 1
  spline S279 degree 3 poles (-13.965032, 1.262518) (-14.143991, 2.083443) (-14.393008, 2.493584) (-15.023506, 2.717124) knots 0 0 0 0 1 1 1 1
  spline S280 degree 3 poles (-20.810093, 28.200141) (-20.961031, 28.845289) (-20.985868, 29.135066) (-20.755322, 29.26371) knots 0 0 0 0 1 1 1 1
  line L51 (-20.755322, 29.26371) -> (-18.396362, 29.26371)
  spline S281 degree 3 poles (-18.396362, 29.26371) (-17.053843, 29.26371) (-15.965435, 30.352118) (-15.965435, 31.69527) knots 0 0 0 0 1 1 1 1
  spline S282 degree 3 poles (-15.965435, 31.69527) (-15.965435, 33.03779) (-17.053843, 34.126829) (-18.396362, 34.126829) knots 0 0 0 0 1 1 1 1
  line L52 (-18.396362, 34.126829) -> (-20.844485, 34.126829)
  spline S283 degree 3 poles (-20.844485, 34.126829) (-20.867412, 34.134467) (-20.889702, 34.140842) (-20.911993, 34.149122) knots 0 0 0 0 1 1 1 1
  spline S284 degree 3 poles (-20.911993, 34.149122) (-16.904181, 37.011842) (-17.332157, 41.608129) (-19.653541, 44.082996) knots 0 0 0 0 1 1 1 1
  spline S285 degree 3 poles (-19.653541, 44.082996) (-21.894681, 46.471889) (-26.113298, 46.736826) (-28.676694, 44.042871) knots 0 0 0 0 1 1 1 1
  spline S286 degree 3 poles (-28.676694, 44.042871) (-30.683467, 41.934201) (-31.624122, 37.485033) (-27.383214, 34.126829) knots 0 0 0 0 1 1 1 1
  line L53 (-27.383214, 34.126829) -> (-29.971448, 34.126829)
  spline S287 degree 3 poles (-29.971448, 34.126829) (-31.313966, 34.126829) (-32.403012, 33.03778) (-32.403012, 31.69527) knots 0 0 0 0 1 1 1 1
  spline S288 degree 3 poles (-32.403012, 31.69527) (-32.403012, 30.352118) (-31.313966, 29.26371) (-29.971448, 29.26371) knots 0 0 0 0 1 1 1 1
  line L54 (-29.971448, 29.26371) -> (-27.681906, 29.26371)
  spline S289 degree 3 poles (-27.681906, 29.26371) (-27.223997, 29.112132) (-27.29469, 28.712816) (-27.564085, 27.651793) knots 0 0 0 0 1 1 1 1
  spline S290 degree 3 poles (-27.564085, 27.651793) (-28.558874, 23.726776) (-29.58869, 19.811944) (-31.133096, 16.059516) knots 0 0 0 0 1 1 1 1
  spline S291 degree 3 poles (-31.133096, 16.059516) (-31.284034, 15.69395) (-31.250917, 15.53346) (-31.087878, 15.446845) knots 0 0 0 0 1 1 1 1
  line L55 (-31.087878, 15.446845) -> (-16.730953, 15.446845)
  spline S292 degree 3 poles (-16.730953, 15.446845) (-16.488306, 15.62644) (-16.599757, 15.857628) (-16.885075, 16.521881) knots 0 0 0 0 1 1 1 1
  spline S293 degree 3 poles (-16.885075, 16.521881) (-18.513545, 20.307427) (-19.866255, 24.185954) (-20.810093, 28.200141) knots 0 0 0 0 1 1 1 1
  spline S294 degree 3 poles (10.928244, 52.757151) (11.430098, 53.66023) (11.470854, 54.618715) (11.181719, 55.577205) knots 0 0 0 0 1 1 1 1
  spline S295 degree 3 poles (11.181719, 55.577205) (10.671586, 57.26618) (9.313785, 58.124679) (7.291089, 58.068636) knots 0 0 0 0 1 1 1 1
  spline S296 degree 3 poles (7.291089, 58.068636) (6.446604, 58.044434) (5.704652, 58.099845) (5.761967, 59.23347) knots 0 0 0 0 1 1 1 1
  spline S297 degree 3 poles (5.761967, 59.23347) (5.790625, 59.805379) (5.38749, 60.020003) (4.94805, 60.021276) knots 0 0 0 0 1 1 1 1
  spline S298 degree 3 poles (4.94805, 60.021276) (2.71901, 60.028919) (0.489971, 59.984975) (-1.739706, 59.971598) knots 0 0 0 0 1 1 1 1
  spline S299 degree 3 poles (-1.739706, 59.971598) (-2.299514, 59.967779) (-2.870148, 59.802828) (-2.88989, 59.232828) knots 0 0 0 0 1 1 1 1
  spline S300 degree 3 poles (-2.88989, 59.232828) (-2.923645, 58.254597) (-3.321049, 57.973105) (-4.226676, 58.138687) knots 0 0 0 0 1 1 1 1
  spline S301 degree 3 poles (-4.226676, 58.138687) (-4.511355, 58.191547) (-4.824058, 58.104296) (-5.121475, 58.073092) knots 0 0 0 0 1 1 1 1
  spline S302 degree 3 poles (-5.121475, 58.073092) (-8.363772, 57.736189) (-9.32226, 54.710427) (-7.821796, 52.190975) knots 0 0 0 0 1 1 1 1
  spline S303 degree 3 poles (-7.821796, 52.190975) (-6.521948, 50.009062) (-5.015116, 47.950706) (-3.597448, 45.838849) knots 0 0 0 0 1 1 1 1
  spline S304 degree 3 poles (-3.597448, 45.838849) (-3.381549, 45.517232) (-3.319773, 45.175869) (-3.344612, 44.788652) knots 0 0 0 0 1 1 1 1
  spline S305 degree 3 poles (-3.344612, 44.788652) (-3.445238, 43.253165) (-3.53822, 41.71831) (-3.598085, 40.18155) knots 0 0 0 0 1 1 1 1
  spline S306 degree 3 poles (-3.598085, 40.18155) (-3.60891, 39.909606) (-3.644577, 39.701352) (-3.744564, 39.552319) knots 0 0 0 0 1 1 1 1
  line L56 (-3.744564, 39.552319) -> (-4.613252, 39.552319)
  spline S307 degree 3 poles (-4.613252, 39.552319) (-5.673638, 39.552319) (-6.53341, 38.693185) (-6.53341, 37.633434) knots 0 0 0 0 1 1 1 1
  spline S308 degree 3 poles (-6.53341, 37.633434) (-6.53341, 36.670494) (-5.824576, 35.876313) (-4.901116, 35.737474) knots 0 0 0 0 1 1 1 1
  spline S309 degree 3 poles (-4.901116, 35.737474) (-4.872458, 35.730467) (-4.846346, 35.720283) (-4.817686, 35.713908) knots 0 0 0 0 1 1 1 1
  line L57 (-4.817686, 35.713908) -> (-4.613252, 35.713908)
  line L58 (-4.613252, 35.713908) -> (7.315292, 35.713908)
  line L59 (7.315292, 35.713908) -> (7.577683, 35.713908)
  spline S310 degree 3 poles (7.577683, 35.713908) (7.959167, 35.787152) (8.276328, 35.933629) (8.521523, 36.14125) knots 0 0 0 0 1 1 1 1
  spline S311 degree 3 poles (8.521523, 36.14125) (8.529167, 36.146342) (8.536173, 36.152717) (8.543816, 36.158441) knots 0 0 0 0 1 1 1 1
  spline S312 degree 3 poles (8.543816, 36.158441) (8.569292, 36.181365) (8.595403, 36.203027) (8.618964, 36.227224) knots 0 0 0 0 1 1 1 1
  spline S313 degree 3 poles (8.618964, 36.227224) (8.997265, 36.577504) (9.234818, 37.076806) (9.234818, 37.633425) knots 0 0 0 0 1 1 1 1
  spline S314 degree 3 poles (9.234818, 37.633425) (9.234818, 38.693175) (8.375046, 39.55231) (7.315296, 39.55231) knots 0 0 0 0 1 1 1 1
  line L60 (7.315296, 39.55231) -> (6.614742, 39.55231)
  spline S315 degree 3 poles (6.614742, 39.55231) (6.540231, 39.647204) (6.499469, 39.777764) (6.492462, 39.960547) knots 0 0 0 0 1 1 1 1
  spline S316 degree 3 poles (6.492462, 39.960547) (6.425589, 41.736774) (6.36254, 43.513001) (6.276566, 45.28795) knots 0 0 0 0 1 1 1 1
  spline S317 degree 3 poles (6.276566, 45.28795) (6.260007, 45.628035) (6.431964, 45.844573) (6.595637, 46.100594) knots 0 0 0 0 1 1 1 1
  spline S318 degree 3 poles (6.595637, 46.100594) (8.016482, 48.334099) (9.639226, 50.437677) (10.928244, 52.757151) knots 0 0 0 0 1 1 1 1
  spline S319 degree 3 poles (70.2691, 19.597325) (69.066692, 22.070282) (68.041975, 24.601197) (67.280913, 27.25822) knots 0 0 0 0 1 1 1 1
  spline S320 degree 3 poles (67.280913, 27.25822) (66.948465, 28.417957) (66.94656, 29.635651) (66.521764, 30.848243) knots 0 0 0 0 1 1 1 1
  line L61 (66.521764, 30.848243) -> (65.264587, 30.848243)
  spline S321 degree 3 poles (65.264587, 30.848243) (64.76783, 30.831052) (64.270432, 30.83423) (63.773676, 30.848243) knots 0 0 0 0 1 1 1 1
  line L62 (63.773676, 30.848243) -> (61.577113, 30.848243)
  spline S322 degree 3 poles (61.577113, 30.848243) (61.216649, 30.79602) (60.847896, 30.827865) (60.48234, 30.848243) knots 0 0 0 0 1 1 1 1
  line L63 (60.48234, 30.848243) -> (59.942271, 30.848243)
  spline S323 degree 3 poles (59.942271, 30.848243) (59.566521, 30.803026) (59.372271, 30.608776) (59.345527, 30.078911) knots 0 0 0 0 1 1 1 1